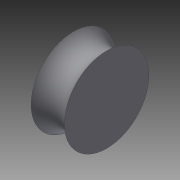
# Autodesk Inventor part: X_Wheel-Rod-Rev1
Saved by Autodesk Inventor 2015 (Build 190159000, 159)
## iProperties
Created: 2016-12-21
Part Number: X_Wheel-Rod-Rev1
Material: Generic
Document SubType Name: Modeling
Designer: Guy
Density: 1 g/cm^3
Appearance: Default
Mass: 57.4891 g
Surface Area: 113.886 cm^2
Volume: 57.4891 cm^3
Author: Guy
Autodesk Inventor part; units mm, degrees
ref_plane "YZ Plane" through (0, 0, 0) normal (1, 0, 0) x (0, 1, 0)
ref_plane "XZ Plane" through (0, 0, 0) normal (0, 1, 0) x (-1, 0, 0)
ref_plane "XY Plane" through (0, 0, 0) normal (0, 0, 1) x (1, 0, 0)
sketch "Sketch2" plane through (0, 0, 0) normal (0, 0, 1) x (1, 0, 0)
  line L0 (-12.5, 0) -> (12.5, 0)
  line L1 (12.5, 0) -> (12.5, -31.7084)
  line L2 (12.5, -31.7084) -> (-12.5, -31.7084)
  line L3 (-12.5, -31.7084) -> (-12.5, 0)
  circle A0 centre (0, -40) radius 15
  point P0 (0, 0)
  point P1 (0, 0)
  dimension "d4" = 25
  dimension "d5" = 30
  dimension "d8" = 40
  constraints: 8 end point, 2 parallel, 2 point on circle, 1 centre point, 1 coincident, 1 horizontal, 1 midpoint, 1 perpendicular
  measures "d4" distance between parallel lines of L1 L3
  measures "d5" diameter of A0
  measures "d8" distance of A0.centre point (0, 0)
revolve "Revolution2" add sketch "Sketch2" angle 360 about axis through (-12.5, 0, 0) along (1, 0, 0) contours L0 L1 A0 L3
body "Solid2"
